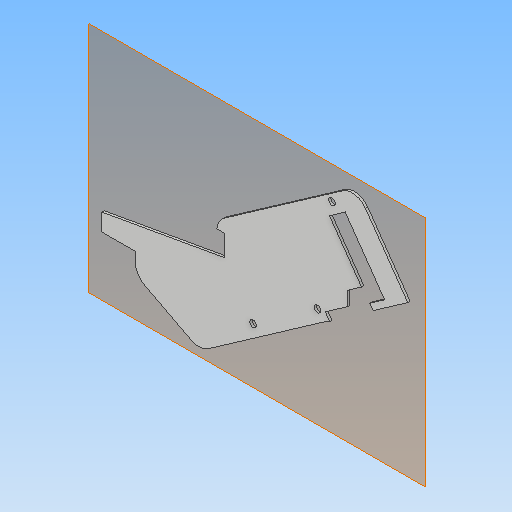
# Autodesk Inventor part: cellSTORM_inverted_opticsmodule_lid
Saved by Autodesk Inventor 2019.4 (Build 234330000, 330)
## iProperties
Created: 2020-11-09
Part Number: cellSTORM_inverted_opticsmodule_lid
Material: Generic
Document SubType Name: Modeling
Designer: diederichbenedict
Density: 1 g/cm^3
Appearance: Default
Author: diederichbenedict
Autodesk Inventor part; units mm, degrees
ref_plane "YZ Plane" through (0, 0, 0) normal (1, 0, 0) x (0, 1, 0)
ref_plane "XZ Plane" through (0, 0, 0) normal (0, 1, 0) x (-1, 0, 0)
ref_plane "XY Plane" through (0, 0, 0) normal (0, 0, 1) x (1, 0, 0)
ref_plane "Work Plane1" through (0, 0, 0) normal (0, 0, 1) x (1, 0, 0)
sketch "Sketch1" plane through (0, 0, 0) normal (0, 0, 1) x (1, 0, 0)
  arc A0 (-7.9352, -23.1681) -> (-8.7998, -28.0716) centre (-7.9352, -25.6961) ccw projected
  line L0 (-8.7998, -28.0716) -> (-27.4567, -41.1353) projected
  arc A1 (-34.704, -41.6104) -> (-27.4567, -41.1353) centre (-31.4718, -35.4013) ccw projected
  line L1 (-34.704, -41.6104) -> (-51.738, -32.743) projected
  arc A2 (-55.5058, -26.5339) -> (-51.738, -32.743) centre (-48.5058, -26.5339) ccw projected
  line L2 (-55.5058, -26.5339) -> (-55.5058, -22.4494) projected
  arc A3 (-49.7326, -15.5577) -> (-55.5058, -22.4494) centre (-48.5058, -22.4494) ccw projected
  line L3 (-49.7326, -15.5577) -> (-17.3058, -9.7854) projected
  line L4 (-17.3058, -9.7854) -> (-7.9352, -23.1681) projected
  line L5 (24.8783, -8.1523) -> (23.0703, -5.7559) projected
  line L6 (23.0703, -5.7559) -> (22.5789, -6.1) projected
  arc A4 (22.5789, -6.1) -> (17.1147, -5.1366) centre (19.7211, -6.3309) ccw projected
  line L7 (17.1147, -5.1366) -> (18.5334, -7.1626) projected
  circle A5 centre (19.7211, -6.3309) radius 1.45 projected
  line L8 (18.5334, -7.1626) -> (19.2274, -8.1539) projected
  line L9 (19.2274, -8.1539) -> (-1.2514, -22.4933) projected
  line L10 (-1.2514, -22.4933) -> (-17.3116, 0.4431) projected
  line L11 (3.5665, 15.0622) -> (-17.3116, 0.4431) projected
  arc A6 (6.3584, 22.4292) -> (3.5665, 15.0622) centre (10.3734, 16.6951) ccw projected
  line L12 (6.3584, 22.4292) -> (14.6012, 28.2009) projected
  arc A7 (24.3503, 26.4818) -> (14.6012, 28.2009) centre (18.6163, 22.4668) ccw projected
  line L13 (24.3503, 26.4818) -> (36.2081, 9.5471) projected
  line L14 (36.2081, 9.5471) -> (39.0496, 11.5367) projected
  line L15 (39.0496, 11.5367) -> (25.5762, 30.7786) projected
  line L16 (25.5762, 30.7786) -> (31.5151, 34.937) projected
  line L17 (31.5151, 34.937) -> (47.862, 11.5912) projected
  line L18 (47.862, 11.5912) -> (41.9232, 7.4328) projected
  line L19 (41.9232, 7.4328) -> (43.6382, 4.9835) projected
  line L20 (43.6382, 4.9835) -> (58.5058, 15.3939) projected
  line L21 (58.5058, 15.3939) -> (40.3386, 41.3393) projected
  arc A8 (40.3386, 41.3393) -> (30.5895, 43.0583) centre (34.6046, 37.3243) ccw projected
  line L22 (30.5895, 43.0583) -> (-20.5271, 7.2661) projected
  arc A9 (-20.5271, 7.2661) -> (-23.5058, 1.8277) centre (-16.512, 1.532) ccw projected
  line L23 (-23.5058, 1.8277) -> (-20.3058, 1.8277) projected
  line L24 (-20.3058, 1.8277) -> (-20.3058, -7.2723) projected
  line L25 (-20.3058, -7.2723) -> (-72.9074, -16.6359) projected
  line L26 (-72.9074, -16.6359) -> (-72.9074, -24.0723) projected
  line L27 (-72.9074, -24.0723) -> (-58.5058, -24.0723) projected
  line L28 (-58.5058, -24.0723) -> (-58.5058, -28.3544) projected
  arc A10 (-58.5058, -28.3544) -> (-54.738, -34.5635) centre (-51.5058, -28.3544) ccw projected
  line L29 (-54.738, -34.5635) -> (-34.4745, -45.112) projected
  arc A11 (-34.4745, -45.112) -> (-27.2272, -44.637) centre (-31.2423, -38.9029) ccw projected
  line L30 (-27.2272, -44.637) -> (23.0703, -9.4182) projected
  arc A12 (27.0854, -8.1523) -> (23.0703, -9.4182) centre (27.0854, -15.1523) ccw projected
  line L31 (24.8783, -8.1523) -> (27.0854, -8.1523) projected
  circle A13 centre (-7.9352, -25.6961) radius 1.45 projected
  circle A14 centre (25.9387, 36.6719) radius 1.45 projected
  line L32 (24.8783, -8.1523) -> (35.6777, -8.1523) projected
  line L33 (35.6777, -8.1523) -> (35.6777, 3.8477) construction
  line L34 (35.6777, 3.8477) -> (95.6777, 3.8477) construction
  line L35 (95.6777, 3.8477) -> (95.6777, 15.3939) projected
  line L36 (95.6777, 15.3939) -> (58.5058, 15.3939) projected
  line L37 (58.5058, 15.3939) -> (43.6382, 4.9835) projected
  line L38 (43.6382, 4.9835) -> (39.0496, 11.5367) projected
  line L39 (39.0496, 11.5367) -> (32.6777, 7.0751) projected
  line L40 (32.6777, 7.0751) -> (32.6777, 0.9712) projected
  line L41 (32.6777, 0.9712) -> (23.0703, -5.7559) projected
  line L42 (23.0703, -5.7559) -> (24.8783, -8.1523) projected
  line L43 (24.9804, -8.4763) -> (23.0739, -5.7534)
  line L44 (23.0739, -5.7534) -> (32.6777, 0.9712)
  line L45 (32.6777, 0.9712) -> (32.6777, 7.0751)
  line L46 (32.6777, 7.0751) -> (39.0496, 11.5367)
  line L47 (39.0496, 11.5367) -> (43.6382, 4.9835)
  line L48 (43.6382, 4.9835) -> (58.5058, 15.3939)
  constraints: 12 end point, 2 collinear, 1 parallel, 1 perpendicular, 1 point on circle, 1 point on line, 1 other
extrude "Extrusion1" add sketch "Sketch1" along normal blind 1 contours A0 L0 A1 L1 A2 L2 A3 L3 L4 | A5 | L43 A12 L30 A11 L29 A10 L28 L27 L26 L25 L24 L23 A9 L22 A8 L21 L20 L19 L18 L17 L16 L15 L14 L13 A7 L12 A6 L11 L10 L9 L8 L7 A4 L6 L5 | L5 L41 L43 | L6 A4 L7 L8 L9 L10 L11 A6 L12 A7 L13 L39 L40 L41 | L15 L16 L17 L18 L38 | A13 | A14
sketch "Sketch2" plane through (0, 0, 1) normal (0, 0, 1) x (1, 0, 0)
  arc A0 (24.9804, -8.4763) -> (23.0703, -9.4182) centre (27.0854, -15.1523) ccw projected
  line L0 (24.9804, -8.4763) -> (23.0739, -5.7534) projected
  line L1 (23.0739, -5.7534) -> (32.6777, 0.9712) projected
  line L2 (32.6777, 0.9712) -> (32.6777, 7.0751) projected
  line L3 (32.6777, 7.0751) -> (39.0496, 11.5367) projected
  line L4 (39.0496, 11.5367) -> (43.6382, 4.9835) projected
  line L5 (43.6382, 4.9835) -> (58.5058, 15.3939) projected
  line L6 (58.5058, 15.3939) -> (40.3386, 41.3393) projected
  arc A1 (40.3386, 41.3393) -> (30.5895, 43.0583) centre (34.6046, 37.3243) ccw projected
  line L7 (30.5895, 43.0583) -> (-20.5271, 7.2661) projected
  arc A2 (-20.5271, 7.2661) -> (-23.5058, 1.8277) centre (-16.512, 1.532) ccw projected
  line L8 (-23.5058, 1.8277) -> (-20.3058, 1.8277) projected
  line L9 (-20.3058, 1.8277) -> (-20.3058, -7.2723) projected
  line L10 (-20.3058, -7.2723) -> (-72.9074, -16.6359) projected
  line L11 (-72.9074, -16.6359) -> (-72.9074, -24.0723) projected
  line L12 (-72.9074, -24.0723) -> (-58.5058, -24.0723) projected
  line L13 (-58.5058, -24.0723) -> (-58.5058, -28.3544) projected
  arc A3 (-58.5058, -28.3544) -> (-54.738, -34.5635) centre (-51.5058, -28.3544) ccw projected
  line L14 (-54.738, -34.5635) -> (-34.4745, -45.112) projected
  arc A4 (-34.4745, -45.112) -> (-27.2272, -44.637) centre (-31.2423, -38.9029) ccw projected
  line L15 (-27.2272, -44.637) -> (23.0703, -9.4182) projected
  circle A5 centre (25.9387, 36.6719) radius 1.45 projected
  circle A6 centre (-7.9352, -25.6961) radius 1.45 projected
  circle A7 centre (19.7211, -6.3309) radius 1.45 projected
  point P0 (0, 0)
extrude "Extrusion2" cut sketch "Sketch2" against normal blind 1 contours A5 | A6 | A7
sketch "Sketch3" plane through (0, 0, 1) normal (0, 0, 1) x (1, 0, 0)
  line L0 (47.862, 11.5912) -> (31.5151, 34.937) projected
  line L1 (31.5151, 34.937) -> (25.5762, 30.7786) projected
  line L2 (41.9232, 7.4328) -> (25.5762, 30.7786) projected
  line L3 (47.862, 11.5912) -> (41.9232, 7.4328) projected
  line L4 (31.6379, 35.6334) -> (48.5584, 11.4684)
  line L5 (48.5584, 11.4684) -> (41.8004, 6.7364)
  line L6 (41.8004, 6.7364) -> (24.8799, 30.9014)
  line L7 (24.8799, 30.9014) -> (31.6379, 35.6334)
  point P0 (0, 0)
  dimension "d4" = 0.5
  constraints: 8 end point, 3 other
  measures "d4" distance between parallel lines of L0 L4
extrude "Extrusion3" cut sketch "Sketch3" against normal through all contours L3 L2 L1 L0 | L4 L5 L6 L7
body "Solid1"
